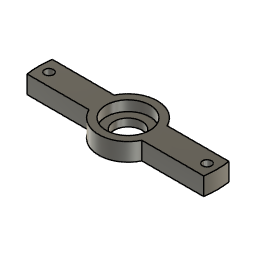
wind_direction_base (Autodesk Fusion 360 design; units mm, degrees)
Autodesk Fusion 360 part; units mm, degrees
note: some values were not read from the file. Set by a fixed rule: which sketch regions a step uses.
sketch "Szkic1" plane through (0, 0, 0) normal (0, 0, 1) x (1, 0, 0)
  circle A0 centre (0, 0) radius 11.5
  circle A1 centre (0, 0) radius 8.6
  circle A2 centre (0, 0) radius 5.5
  dimension "d1" = 23
  dimension "d2" = 17.2
  dimension "d7" = 11
  constraint coincident A0.centre A1.centre
  measures "d1" diameter of A0
  measures "d2" diameter of A1
  measures "d7" diameter of A2
extrude "Wyciągnięcie proste1" add sketch "Szkic1" along normal blind 7 contours A0
extrude "Wyciągnięcie proste2" add sketch "Szkic1" along normal blind 3 contours A1
sketch "Szkic2" plane through (0, 0, 0) normal (0, 0, 1) x (1, 0, 0)
  line L0 (13.1003, -4.95) -> (-13.365, -4.95)
  line L1 (-13.365, -4.95) -> (-13.365, 5.05)
  line L2 (-13.365, 5.05) -> (13.635, 5.05)
  line L3 (13.1003, -4.95) -> (-13.365, 5.05) construction
  line L4 (-13.365, -4.95) -> (13.635, 5.05) construction
  line L5 (35, -4.95) -> (-35, -4.95)
  line L6 (-35, -4.95) -> (-35, 4.95)
  line L7 (-35, 4.95) -> (35, 4.95)
  line L8 (35, 4.95) -> (35, -4.95)
  line L9 (35, -4.95) -> (-35, 4.95) construction
  line L10 (-13.365, -4.95) -> (-21.365, -4.95)
  line L11 (-21.365, -4.95) -> (-21.365, 4.95)
  line L12 (-21.365, 4.95) -> (-13.365, 4.95)
  line L13 (-13.365, 4.95) -> (-13.365, -4.95)
  circle A0 centre (0, 0) radius 11.5
  line L14 (-35, -4.95) -> (-11.3867, -1.6104) construction
  line L15 (0, 0) -> (35, 4.95) construction
  line L16 (-18.365, 4.95) -> (-18.365, -4.95)
  circle A1 centre (0, 0) radius 35
  circle A2 centre (-31, 0) radius 1.75
  circle A3 centre (31, 0) radius 1.75
  dimension "d8" = 27
  dimension "d9" = 10
  dimension "d10" = 70
  dimension "d11" = 9.9
  dimension "d12" = 8
  dimension "d15" = 3
  dimension "d36" = 3.5
  dimension "d37" = 4
  dimension "d38" = 4
  constraint horizontal L0
  constraint perpendicular L0 L1
  constraint parallel L0 L2
  constraint coincident L3 A0.centre
  constraint coincident L4 A0.centre
  constraint coincident A0.centre L15.start
  constraint horizontal L5
  constraint perpendicular L5 L6
  constraint parallel L5 L7
  constraint parallel L6 L8
  constraint coincident L9 A0.centre
  constraint coincident A0.centre L14
  constraint horizontal L10
  constraint vertical L11
  constraint horizontal L12
  constraint vertical L13
  constraint coincident A0 L14.end
  constraint collinear L14 L15
  constraint coincident L7 L16.start
  constraint coincident L12 L16.start
  constraint coincident L10 L16.end
  constraint coincident L5 L16.end
  constraint perpendicular L7 L16
  constraint tangent L8 A1
  constraint horizontal A0.centre A2.centre
  constraint horizontal A0.centre A3.centre
  constraint equal A2 A3
  measures "d8" distance of L1.end L2.end
  measures "d9" distance of L0.end L1.end
  measures "d10" distance of L6.end L7.end
  measures "d11" distance of L5.end L6.end
  measures "d12" distance of L0.end L10.end
  measures "d15" distance of L11 L16
  measures "d36" diameter of A3
  measures "d37" distance of L8 A3.centre
  measures "d38" distance of L6 A2.centre
extrude "Wyciągnięcie proste3" add sketch "Szkic2" along normal blind 7 contours L0 L5 L7 A0 A1 | L0 L1 L5 L7 L13 A0 | L5 L7 L11 A1 | L1 L5 L7 L10 L12 L13 L16 | L5 L7 L10 L11 L12 L16
